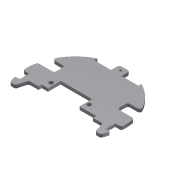
# Autodesk Inventor part: OpenROV_Dev_EChassis_Servo_Plate
Saved by Autodesk Inventor 2012 (Build 160160000, 160)
## iProperties
Created: 2012-08-06
Part Number: OpenROV_Dev_EChassis_Servo_Plate
Material: Default
Document SubType Name: Modeling
Designer: user
Density: 1 g/cm^3
Author: user
Autodesk Inventor part; units mm, degrees
ref_plane "YZ Plane" through (0, 0, 0) normal (1, 0, 0) x (0, 1, 0)
ref_plane "XZ Plane" through (0, 0, 0) normal (0, 1, 0) x (-1, 0, 0)
ref_plane "XY Plane" through (0, 0, 0) normal (0, 0, 1) x (1, 0, 0)
sketch "Sketch1" plane through (0, 0, 0) normal (0, 0, 1) x (1, 0, 0)
  line L0 (-20, 6) -> (10, 6)
  line L1 (10, 6) -> (10, -6)
  line L2 (-20, -6) -> (-20, 6)
  line L3 (-41.6653, -19) -> (-39.523, -19)
  line L4 (-37.5912, -17.5176) -> (-35.7061, -10.4824)
  line L5 (41.6653, -19) -> (39.523, -19)
  line L6 (37.5912, -17.5176) -> (35.7061, -10.4824)
  circle A0 centre (-23.1, 0) radius 2
  circle A1 centre (13.1, 0) radius 2
  line L7 (-26, -9) -> (-26, -6)
  line L8 (26, -9) -> (26, -6)
  line L9 (-26, -6) -> (-20, -6)
  line L10 (10, -6) -> (26, -6)
  line L11 (-33.7742, -9) -> (-26, -9)
  line L12 (26, -9) -> (33.7742, -9)
  arc A2 (-43.5171, -17.7556) -> (-41.6653, -19) centre (-41.6653, -17) ccw
  arc A3 (-39.523, -19) -> (-37.5912, -17.5176) centre (-39.523, -17) ccw
  arc A4 (-33.7742, -9) -> (-35.7061, -10.4824) centre (-33.7742, -11) ccw
  arc A5 (35.7061, -10.4824) -> (33.7742, -9) centre (33.7742, -11) ccw
  arc A6 (37.5912, -17.5176) -> (39.523, -19) centre (39.523, -17) ccw
  arc A7 (41.6653, -19) -> (43.5171, -17.7556) centre (41.6653, -17) ccw
  line L13 (-21, 42.0476) -> (-21, 39.0476)
  line L14 (21, 42.0476) -> (21, 39.0476)
  line L15 (-5, 39.0476) -> (-5, 44.8999)
  line L16 (5, 39.0476) -> (5, 44.8999)
  arc A8 (3.1333, 46.8954) -> (-3.1333, 46.8954) centre (0, 0) ccw
  line L17 (-21, 39.0476) -> (-5, 39.0476)
  line L18 (5, 39.0476) -> (21, 39.0476)
  circle A9 centre (0, 43.0476) radius 1
  arc A10 (-3.1333, 46.8954) -> (-5, 44.8999) centre (-3, 44.8999) ccw
  arc A11 (5, 44.8999) -> (3.1333, 46.8954) centre (3, 44.8999) ccw
  line L19 (44.9889, -3) -> (41, -3)
  line L20 (41, -3) -> (41, -12)
  line L21 (41, -12) -> (44.1248, -12)
  arc A12 (43.5171, -17.7556) -> (45.0841, -13.2826) centre (0, 0) ccw
  line L22 (-44.9889, -3) -> (-41, -3)
  line L23 (-41, -3) -> (-41, -12)
  line L24 (-41, -12) -> (-44.1248, -12)
  arc A13 (-45.0841, -13.2826) -> (-43.5171, -17.7556) centre (0, 0) ccw
  line L25 (-39.2556, 20) -> (-32, 20)
  line L26 (-30, 18) -> (-30, 12)
  line L27 (-32, 10) -> (-44.2832, 10)
  line L28 (32, 20) -> (39.2556, 20)
  line L29 (44.2832, 10) -> (32, 10)
  line L30 (30, 12) -> (30, 18)
  arc A14 (46.9884, -1.0444) -> (46.2513, 8.3556) centre (0, 0) ccw
  arc A15 (41.0003, 22.9778) -> (21, 42.0476) centre (0, 0) ccw
  arc A16 (-21, 42.0476) -> (-41.0003, 22.9778) centre (0, 0) ccw
  arc A17 (-46.2513, 8.3556) -> (-46.9884, -1.0444) centre (0, 0) ccw
  arc A18 (39.2556, 20) -> (41.0003, 22.9778) centre (39.2556, 22) ccw
  arc A19 (46.2513, 8.3556) -> (44.2832, 10) centre (44.2832, 8) ccw
  arc A20 (-41.0003, 22.9778) -> (-39.2556, 20) centre (-39.2556, 22) ccw
  arc A21 (-44.2832, 10) -> (-46.2513, 8.3556) centre (-44.2832, 8) ccw
  arc A22 (32, 20) -> (30, 18) centre (32, 18) ccw
  arc A23 (30, 12) -> (32, 10) centre (32, 12) ccw
  arc A24 (-30, 18) -> (-32, 20) centre (-32, 18) ccw
  arc A25 (-32, 10) -> (-30, 12) centre (-32, 12) ccw
  arc A26 (-44.1248, -12) -> (-45.0841, -13.2826) centre (-44.1248, -13) ccw
  arc A27 (45.0841, -13.2826) -> (44.1248, -12) centre (44.1248, -13) ccw
  arc A28 (-46.9884, -1.0444) -> (-44.9889, -3) centre (-44.9889, -1) ccw
  arc A29 (44.9889, -3) -> (46.9884, -1.0444) centre (44.9889, -1) ccw
  point P0 (-35.3089, -9)
  point P1 (35.3089, -9)
  point P2 (-42.9884, -19)
  point P3 (-37.9884, -19)
  point P4 (42.9884, -19)
  point P5 (37.9884, -19)
  point P6 (-5, 46.7333)
  point P7 (5, 46.7333)
  point P8 (46.9042, -3)
  point P9 (45.4423, -12)
  point P10 (-46.9042, -3)
  point P11 (-45.4423, -12)
  point P12 (-42.5323, 20)
  point P13 (-45.9239, 10)
  point P14 (45.9239, 10)
  point P15 (42.5323, 20)
  dimension "d1" = 30
  dimension "d2" = 12
  dimension "d3" = 10
  dimension "d4" = 6
  dimension "d8" = 5
  dimension "d11" = 5
  dimension "d17" = 4
  dimension "d18" = 4
  dimension "d19" = 36.2
  dimension "d20" = 3.1
  dimension "d31" = 52
  dimension "d51" = 2
  dimension "d58" = 12
  dimension "d59" = 3
  dimension "d60" = 3
  dimension "d89" = 42
  dimension "d93" = 10
  dimension "d94" = 5
  dimension "d95" = 2
  dimension "d96" = 4
  dimension "d99" = 2
  dimension "d101" = 9
  dimension "d103" = 9
  dimension "d106" = 47
  dimension "d107" = 47
  dimension "d108" = 10
  dimension "d109" = 30
  dimension "d110" = 10
  dimension "d111" = 10
  dimension "d112" = 30
  dimension "d113" = 2
  dimension "d114" = 41
  dimension "d115" = 41
  dimension "d116" = 1
  dimension "d117" = 2
  constraints: 64 point on circle, 62 end point, 38 tangent, 30 centre point, 20 point on line, 15 equal radius, 12 parallel, 9 perpendicular, 3 horizontal, 2 collinear
  measures "d1" distance of L0.start L0.end
  measures "d2" distance of L2.start L0.start
  measures "d3" distance from line of point (0, 0) L1
  measures "d4" distance from line of point (0, 0) L0
  measures "d8" distance of point (-42.988, -19) point (-37.988, -19)
  measures "d11" distance of point (42.988, -19) point (37.988, -19)
  measures "d17" diameter of A0
  measures "d18" diameter of A1
  measures "d19" distance of A1.centre A0.centre
  measures "d20" distance from line of L2 A0.centre
  measures "d31" distance between parallel lines of L8 L7
  measures "d51" radius of A2
  measures "d58" distance between parallel lines of L10 L0
  measures "d59" distance between parallel lines of L12 L10
  measures "d60" distance between parallel lines of L11 L9
  measures "d89" distance of L13.start L14.start
  measures "d93" distance between parallel lines of L16 L15
  measures "d94" distance from line of point (0, 0) L15
  measures "d95" diameter of A9
  measures "d96" distance from line of L17 A9.centre
  measures "d99" radius of A10
  measures "d101" distance of L19.end L20.end
  measures "d103" distance of L22.end L23.end
  measures "d106" radius of A13
  measures "d107" radius of A12
  measures "d108" distance between parallel lines of L27 L25
  measures "d109" distance from line of point (0, 0) L26
  measures "d110" distance from line of point (0, 0) L27
  measures "d111" distance from line of point (0, 0) L29
  measures "d112" distance from line of point (0, 0) L30
  measures "d113" radius of A18
  measures "d114" distance from line of point (0, 0) L23
  measures "d115" distance from line of point (0, 0) L20
  measures "d116" radius of A26
  measures "d117" radius of A28
extrude "Extrusion3" add sketch "Sketch1" along normal blind 3
body "Solid3"
